MetalHornCalibrationNeedle (Autodesk Fusion 360 design; units mm, degrees)
Autodesk Fusion 360 part; units mm, degrees
note: some values were not read from the file. Set by a fixed rule: which sketch regions a step uses.
sketch "Sketch1" plane through (0, 0, 0) normal (0, 1, 0) x (1, 0, 0)
  circle A0 centre (0, 0) radius 10.75
  line L0 (-9.8524, 4.3003) -> (-3, 20)
  line L1 (-3, 20) -> (3, 20)
  line L2 (3, 20) -> (9.8524, 4.3003)
  line L3 (0, 0) -> (0, 20) construction
  line L4 (3, 20) -> (0.75, 70)
  line L5 (0.75, 70) -> (-0.75, 70)
  line L6 (-0.75, 70) -> (-3, 20)
  line L7 (0, 20) -> (0, 70) construction
  dimension "d1" = 21.5
  dimension "d6" = 6
  dimension "d7" = 20
  dimension "d8" = 90
  dimension "d14" = 90
  dimension "d15" = 1.5
  dimension "d16" = 70
  constraint coincident A0.centre L3.start
  constraint coincident A0 L0.start
  constraint horizontal L1
  constraint coincident A0 L2.end
  constraint tangent A0 L2
  constraint tangent A0 L0
  constraint midpoint L1 L3.end
  constraint parallel L1 L5
  constraint midpoint L5 L7.end
  measures "d1" diameter of A0
  measures "d6" distance of L0.end L1.end
  measures "d7" distance of A0.centre L1
  measures "d8" angle of L1 L3
  measures "d14" angle of L5 L7
  measures "d15" distance of L4.end L5.end
  measures "d16" distance of A0.centre L5
extrude "Extrude1" add sketch "Sketch1" along normal blind 2
sketch "Sketch2" plane through (0, 2, 0) normal (0, 1, 0) x (-1, 0, 0)
  arc A0 (9.8524, -4.3003) -> (-9.8524, -4.3003) centre (0, 0) ccw
  circle A1 centre (0, 0) radius 7
  line L0 (-9.8524, -4.3003) -> (-3, -20)
  line L1 (3, -20) -> (9.8524, -4.3003)
  line L2 (0, 0) -> (0, -7) construction
  circle A2 centre (0, -7) radius 1.75
  circle A3 centre (7, 0) radius 1.75
  circle A4 centre (0, 7) radius 1.75
  circle A5 centre (-7, 0) radius 1.75
  line L3 (-3, -20) -> (-0.75, -70)
  line L4 (-0.75, -70) -> (0.75, -70)
  line L5 (0.75, -70) -> (3, -20)
  dimension "d5" = 14
  dimension "d9" = 3.5
  dimension "d11" = 360
  constraint concentric A0 A1
  constraint coincident A0.centre A1.centre
  constraint coincident A1 L2.end
  constraint vertical L2
  constraint coincident L2.end A2.centre
  measures "d5" diameter of A1
  measures "d9" diameter of A2
extrude "Extrude2" cut sketch "Sketch2" against normal up to surface (2 mm away) contours A1 A3 | A1 A3 | A1 A4 | A1 A4 | A1 A2 | A1 A2 | A1 A5 | A1 A5
sketch "Sketch4" plane through (0, 2, 0) normal (0, 1, 0) x (-1, 0, 0)
  circle A0 centre (7, 0) radius 1.75
  circle A1 centre (0, 7) radius 1.75
  circle A2 centre (0, -7) radius 1.75
  circle A3 centre (-7, 0) radius 1.75
  line L0 (-3, -20) -> (-0.75, -70)
  line L1 (-0.75, -70) -> (0.75, -70)
  line L2 (0.75, -70) -> (3, -20)
  line L3 (3, -20) -> (9.8524, -4.3003)
  arc A4 (9.8524, -4.3003) -> (-9.8524, -4.3003) centre (0, 0) ccw
  line L4 (-9.8524, -4.3003) -> (-3, -20)
  circle A5 centre (0, 0) radius 10.75 construction
  constraint concentric A4 A5
  constraint coincident L3.end A5
sketch "Sketch3" plane through (0, 0, 0) normal (1, 0, 0) x (0, 0, -1)
  line L0 (-1.75, 2) -> (1.75, 2)
  line L1 (-8.75, 2) -> (-5.25, 2)
  line L2 (5.25, 2) -> (8.75, 2)
  line L3 (-1.75, 2) -> (1.75, 2)
  line L4 (20, 2) -> (70, 2)
  line L5 (70, 2) -> (20, 2)
  line L6 (20, 2) -> (4.3003, 2)
  line L7 (4.3003, 2) -> (-10.75, 2)
  line L8 (4.3003, 2) -> (20, 2)
  line L9 (10.75, 2) -> (-10.75, 2)
  line L10 (20.75, 2) -> (19.25, 2)
  line L11 (19.25, 2) -> (19.25, 10)
  line L12 (19.25, 10) -> (20.75, 10)
  line L13 (20.75, 10) -> (20.75, 2)
  line L14 (20, 10) -> (20, 2) construction
  dimension "d17" = 1.5
  dimension "d18" = 8
  constraint horizontal L10
  constraint vertical L11
  constraint horizontal L12
  constraint vertical L13
  constraint coincident L5 L10.start
  constraint midpoint L12 L14.start
  constraint midpoint L10 L4.start
  constraint coincident L4.start L14
  measures "d17" distance of L11.end L12.end
  measures "d18" distance of L10.end L11.end
extrude "Extrude3" add sketch "Sketch3" along normal up to surface end surface through (-9.8524, 0, -4.3003) normal (-0.916505, 0, -0.400024) offset 0
mirror "Mirror1" about plane through (0, 0, 0) normal (1, 0, 0) of "Extrude3"
sketch "Sketch5" plane through (0, 2, 0) normal (0, 1, 0) x (-1, 0, 0)
  line L0 (-2.6726, -20.75) -> (-3, -20)
  line L1 (-3, -20) -> (-0.75, -70)
  line L2 (-0.75, -70) -> (0.75, -70)
  line L3 (0.75, -70) -> (3, -20)
  line L4 (3, -20) -> (2.6726, -20.75)
  line L5 (2.6726, -20.75) -> (-2.6726, -20.75)
  line L6 (2.6726, -20.75) -> (3.3274, -19.25)
  line L7 (3.3274, -19.25) -> (-3.3274, -19.25)
  line L8 (-3.3274, -19.25) -> (-2.6726, -20.75)
  line L9 (-2.6726, -20.75) -> (2.6726, -20.75)
  line L10 (2.6726, -20.75) -> (2.9663, -20.75)
  line L11 (-2.6726, -20.75) -> (-2.9663, -20.75)
  line L12 (0.75, -70) -> (-0.75, -70)
  line L13 (-0.75, -70) -> (-0.75, -20.75)
  line L14 (-0.75, -20.75) -> (0.75, -20.75)
  line L15 (0.75, -20.75) -> (0.75, -70)
  circle A0 centre (7, 0) radius 1.75
  circle A1 centre (0, 7) radius 1.75
  circle A2 centre (0, -7) radius 1.75
  circle A3 centre (-7, 0) radius 1.75
  line L16 (-3.3274, -19.25) -> (3.3274, -19.25)
  line L17 (3.3274, -19.25) -> (9.8524, -4.3003)
  arc A4 (9.8524, -4.3003) -> (-9.8524, -4.3003) centre (0, 0) ccw
  line L18 (-9.8524, -4.3003) -> (-3.3274, -19.25)
  circle A5 centre (0, 0) radius 10.75
  constraint coincident L4.end L5.start
  constraint coincident L3 L10.end
  constraint parallel L9 L10
  constraint coincident L0.start L5.end
  constraint coincident L1 L11.end
  constraint parallel L5 L11
  constraint horizontal L12
  constraint vertical L13
  constraint horizontal L14
  constraint vertical L15
  constraint coincident L9 L13.end
  constraint coincident L2.end L3.start
  constraint coincident L1.end L2.start
  constraint concentric A4 A5
  constraint coincident L17.end A5
extrude "Extrude4" add sketch "Sketch5" along normal up to surface (8 mm away) contours L0 L1 L8 L11 | L2 L5 L9 L12 L13 L14 L15 | L7 L16 L17 L18 A5 | L3 L4 L6 L10
sketch "Sketch6" plane through (0, 0, 0) normal (1, 0, 0) x (0, 0, -1)
  line L0 (20, 10) -> (20, 0)
  line L1 (20, 0) -> (4.3003, 0)
  line L2 (4.3003, 0) -> (4.3003, 2)
  line L3 (4.3003, 2) -> (4.3003, 10)
  line L4 (4.3003, 10) -> (20, 10)
  line L5 (70, 0) -> (20, 0)
  line L6 (20, 0) -> (20, 10)
  line L7 (20, 10) -> (20.75, 10)
  line L8 (20.75, 10) -> (20.75, 2)
  line L9 (20.75, 2) -> (70, 2)
  line L10 (70, 2) -> (70, 0)
  line L11 (20.75, 10) -> (70, 10)
  line L12 (70, 10) -> (70, 2)
  line L13 (70, 2) -> (20.75, 2)
  line L14 (20.75, 2) -> (20.75, 10)
  line L15 (4.3003, 0) -> (-10.75, 0)
  line L16 (4.3003, 0) -> (4.3003, 2)
  line L17 (4.3003, 2) -> (-10.75, 2)
  line L18 (4.3003, 2) -> (4.3003, 0)
  line L19 (10.75, 10) -> (4.3003, 10)
  line L20 (4.3003, 10) -> (4.3003, 2)
  line L21 (10.75, 2) -> (4.3003, 2)
  line L22 (4.3003, 2) -> (4.3003, 10)
  line L23 (8.75, 0) -> (5.25, 0)
  line L24 (5.25, 2) -> (8.75, 2)
  line L25 (7, 2) -> (7, 4.5)
  line L26 (7, 4.5) -> (18, 10)
  point P0 (7, 2)
  dimension "d25" = 2.5
  dimension "d26" = 2
  constraint coincident P0 L25.start
  constraint perpendicular L24 L25
  constraint coincident L4 L26.end
  measures "d25" distance of P0 L25.end
  measures "d26" distance of L0.start L26.end
extrude "Extrude5" cut sketch "Sketch6" against normal through all contours L3 L4 L19 L20 L21 L22 L24 L25 L26
mirror "Mirror2" about plane through (0, 0, 0) normal (1, 0, 0) of "Extrude5"
sketch "Sketch7" plane through (0, 0, 0) normal (1, 0, 0) x (0, 0, -1)
  line L0 (70, 10) -> (20.75, 10)
  line L1 (20.75, 10) -> (20.75, 2)
  line L2 (20.75, 2) -> (70, 2)
  line L3 (70, 2) -> (70, 10)
  line L4 (20, 0) -> (70, 0)
  line L5 (70, 0) -> (70, 2)
  line L6 (70, 2) -> (20.75, 2)
  line L7 (20.75, 2) -> (20.75, 10)
  line L8 (20.75, 10) -> (20, 10)
  line L9 (20, 10) -> (20, 0)
  line L10 (70, 7.5) -> (62.5, 0)
  dimension "d30" = 2.5
  dimension "d31" = 45
  constraint coincident L3 L10.start
  constraint coincident L4 L10.end
  measures "d30" distance of L0.start L10.start
  measures "d31" angle of L3 L10
extrude "Extrude6" cut sketch "Sketch7" along normal through all contours L2 L3 L6 L10 | L2 L4 L5 L6 L10
mirror "Mirror3" about plane through (0, 0, 0) normal (1, 0, 0) of "Extrude6"
chamfer "Chamfer1" distance 2 angle 45 6 edges at (0.75, 6, -20.75) (0.75, 2, -42.625) (1.8581, 2, -20.75) (-0.75, 6, -20.75) (-1.8581, 2, -20.75) (-0.75, 2, -42.625)
chamfer "Chamfer2" distance 0.5 angle 45 2 edges at (-0.75, 8.75, -70) (0.75, 8.75, -70)
sketch "Sketch8" plane through (0, 2, 0) normal (0, 1, 0) x (-1, 0, 0)
  circle A0 centre (0, -7) radius 1.75
  arc A1 (-8.1586, -7) -> (8.1586, -7) centre (0, 0) ccw
  line L0 (8.1586, -7) -> (8.6741, -7)
  line L1 (8.6741, -7) -> (9.8524, -4.3003)
  arc A2 (9.8524, -4.3003) -> (-9.8524, -4.3003) centre (0, 0) ccw
  line L2 (-9.8524, -4.3003) -> (-8.6741, -7)
  line L3 (-8.6741, -7) -> (-8.1586, -7)
  circle A3 centre (7, 0) radius 1.75
  circle A4 centre (0, 7) radius 1.75
  circle A5 centre (-7, 0) radius 1.75
  circle A6 centre (0, 0) radius 3
  dimension "d37" = 6
  constraint coincident A1.centre A2.centre
  measures "d37" diameter of A6
extrude "Extrude7" cut sketch "Sketch8" against normal up to surface (2 mm away) contours A6
equation "d14 = d8"
